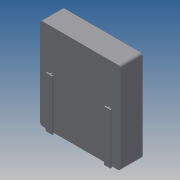
# Autodesk Inventor part: Insert
Saved by Autodesk Inventor 2014 (Build 180170000, 170)
## iProperties
Created: 2014-05-15
Part Number: Insert
Material: Generic
Document SubType Name: Modeling
Designer: 1770749
Density: 1 g/cm^3
Appearance: Default
Author: 1770749
Autodesk Inventor part; units mm, degrees
ref_plane "YZ Plane" through (0, 0, 0) normal (1, 0, 0) x (0, 1, 0)
ref_plane "XZ Plane" through (0, 0, 0) normal (0, 1, 0) x (-1, 0, 0)
ref_plane "XY Plane" through (0, 0, 0) normal (0, 0, 1) x (1, 0, 0)
sketch "Sketch1" plane through (0, 0, 0) normal (0, 1, 0) x (-1, 0, 0)
  line L0 (0, 0) -> (62, 0)
  line L1 (62, 0) -> (62, 70)
  line L2 (62, 70) -> (0, 70)
  line L3 (0, 70) -> (0, 0)
  dimension "d0" = 62
  dimension "d1" = 70
  constraints: 8 end point, 2 parallel, 1 horizontal, 1 perpendicular
  measures "d0" distance of L2.end L1.end
  measures "d1" distance of L1.end L0.end
extrude "Extrusion1" add sketch "Sketch1" along normal blind 2
sketch "Sketch2" plane through (0, 2, 0) normal (0, 1, 0) x (1, 0, 0)
  line L0 (0, 0) -> (-62, 0) projected
  line L1 (-62, 0) -> (-62, -70) projected
  line L2 (-62, -70) -> (0, -70) projected
  line L3 (0, -70) -> (0, 0) projected
  line L4 (-60, -2) -> (-2, -2)
  line L5 (-2, -2) -> (-2, -68)
  line L6 (-2, -68) -> (-60, -68)
  line L7 (-60, -68) -> (-60, -2)
  line L8 (0, 0) -> (-62, 0) projected
  line L9 (-62, 0) -> (-62, -70) projected
  line L10 (-62, -70) -> (0, -70) projected
  line L11 (0, -70) -> (0, 0) projected
  dimension "d4" = 2
  dimension "d5" = 2
  dimension "d6" = 2
  dimension "d7" = 2
  constraints: 8 end point, 2 parallel, 1 horizontal, 1 perpendicular
  measures "d4" distance between parallel lines of L0 L4
  measures "d5" distance between parallel lines of L1 L7
  measures "d6" distance between parallel lines of L2 L6
  measures "d7" distance between parallel lines of L3 L5
extrude "Extrusion2" add sketch "Sketch2" along normal blind 15
fillet "Fillet1" radius 2 4 edges at (-62, 8.5, 70) (-62, 8.5, 0) (0, 8.5, 0) (0, 8.5, 70)
sketch "Sketch3" plane through (-2, 0, 0) normal (0, 0, -1) x (-1, 0, 0)
  line L0 (0, 0) -> (58, 0) projected
  line L1 (8.7434, -1) -> (3.7434, -1)
  line L2 (3.7434, -1) -> (3.7434, -2)
  line L3 (3.7434, -2) -> (8.7434, -2)
  line L4 (8.7434, -2) -> (8.7434, -1)
  line L5 (5.7434, 0) -> (6.7434, 0)
  line L6 (6.7434, 0) -> (6.7434, -1)
  line L7 (6.7434, -1) -> (5.7434, -1)
  line L8 (5.7434, -1) -> (5.7434, 0)
  line L9 (50.59, 0) -> (51.59, 0)
  line L10 (51.59, 0) -> (51.59, -1)
  line L11 (51.59, -1) -> (50.59, -1)
  line L12 (50.59, -1) -> (50.59, 0)
  line L13 (48.59, -1) -> (53.59, -1)
  line L14 (53.59, -1) -> (53.59, -2)
  line L15 (53.59, -2) -> (48.59, -2)
  line L16 (48.59, -2) -> (48.59, -1)
  point P0 (-2, 0)
  point P1 (29, 0)
  point P2 (9.41, 0)
  point P3 (48.59, 0)
  dimension "d11" = 19.59
  dimension "d12" = 19.59
  dimension "d14" = 2
  dimension "d15" = 2
  dimension "d16" = 2
  dimension "d17" = 2
  dimension "d18" = 2
  dimension "d19" = 1
  dimension "d20" = 1
  dimension "d21" = 1
  dimension "d22" = 1
  dimension "d23" = 1
  dimension "d24" = 1
  constraints: 32 end point, 8 parallel, 5 point on line, 4 horizontal, 4 perpendicular, 1 midpoint
  measures "d11" distance of point (9.41, 0) point (29, 0)
  measures "d12" distance of point (48.59, 0) point (29, 0)
  measures "d14" distance from line of L1.end L8
  measures "d15" horizontal distance of L1.start L5.end
  measures "d16" distance of L11.end L13.start
  measures "d17" distance of L9.start point (48.59, 0)
  measures "d18" distance of L13.end L10.end
  measures "d19" distance of L9.end L9.start
  measures "d20" distance between parallel lines of L1 L3
  measures "d21" distance of L13.end L14.end
  measures "d22" distance of L5.end L6.end
  measures "d23" distance of L5.start L5.end
  measures "d24" distance of L9.end L10.end
extrude "Extrusion3" add sketch "Sketch3" against normal blind 39
body "Solid1"
